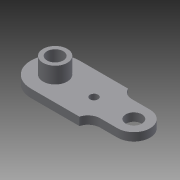
# Autodesk Inventor part: 4-3
Saved by Autodesk Inventor 2015 SP2 (Build 190223200, 223)
## iProperties
Created: 2015-09-16
Part Number: 4-3
Material: Generic
Document SubType Name: Modeling
Designer: Brandon
Density: 1 g/cm^3
Appearance: Default
Author: Brandon
Autodesk Inventor part; units mm, degrees
ref_plane "YZ Plane" through (0, 0, 0) normal (1, 0, 0) x (0, 1, 0)
ref_plane "XZ Plane" through (0, 0, 0) normal (0, 1, 0) x (-1, 0, 0)
ref_plane "XY Plane" through (0, 0, 0) normal (0, 0, 1) x (1, 0, 0)
sketch "Sketch1" plane through (0, 0, 0) normal (0, 0, 1) x (1, 0, 0)
  circle A0 centre (0, 0) radius 15
  circle A1 centre (0, 0) radius 10
  circle A2 centre (0, 0) radius 30
  circle A3 centre (95.994, 1.0738) radius 10
  circle A4 centre (95.994, 1.0738) radius 20
  circle A5 centre (48, 0) radius 5
  line L0 (96, -18.9262) -> (74.477, -18.9262)
  line L1 (0, -30) -> (60, -30)
  arc A6 (74.477, -18.9262) -> (60, -30) centre (74.477, -33.9262) ccw
  line L2 (0, 30) -> (60, 30)
  line L3 (95.994, 21.0738) -> (73.7153, 21.0738)
  arc A7 (60, 30) -> (73.7153, 21.0738) centre (73.7153, 36.0738) ccw
  dimension "d0" = 30
  dimension "d1" = 20
  dimension "d2" = 60
  dimension "d6" = 20
  dimension "d7" = 40
  dimension "d8" = 10
  dimension "d9" = 48
  dimension "d10" = 96
  dimension "d11" = 60
  dimension "d12" = 30
  dimension "d13" = 60
  dimension "d14" = 30
  constraints: 8 centre point, 8 end point, 8 point on circle, 4 coincident, 4 horizontal, 4 tangent
  measures "d0" diameter of A0
  measures "d1" diameter of A1
  measures "d2" diameter of A2
  measures "d6" diameter of A3
  measures "d7" diameter of A4
  measures "d8" diameter of A5
  measures "d9" distance of point (0, 0) A5.centre
  measures "d10" distance of A3.centre point (0, 0)
  measures "d11" distance of L1.start L1.end
  measures "d12" diameter of A6
  measures "d13" distance of L2.start L2.end
  measures "d14" diameter of A7
extrude "Extrusion1" add sketch "Sketch1" along normal blind 10 contours A0 | A2 | A4 | A2 L2 A7 L3 A4 L0 A6 L1
sketch "Sketch2" plane through (0, 0, 10) normal (0, 0, 1) x (1, 0, 0)
  circle A0 centre (0, 0) radius 10
  circle A1 centre (0, 0) radius 15
  dimension "d17" = 20
  dimension "d18" = 30
  constraints: 2 centre point, 2 coincident
  measures "d17" diameter of A0
  measures "d18" diameter of A1
extrude "Extrusion2" add sketch "Sketch2" along normal blind 20
body "Solid1"
